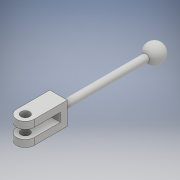
# Autodesk Inventor part: EndJoint
Saved by Autodesk Inventor 2018 (Build 220112000, 112)
## iProperties
Created: 2017-06-01
Part Number: EndJoint
Material: Generic
Document SubType Name: Modeling
Designer: Damian
Density: 1 g/cm^3
Appearance: Default
Author: Damian
Autodesk Inventor part; units mm, degrees
ref_plane "YZ Plane" through (0, 0, 0) normal (1, 0, 0) x (0, 1, 0)
ref_plane "XZ Plane" through (0, 0, 0) normal (0, 1, 0) x (-1, 0, 0)
ref_plane "XY Plane" through (0, 0, 0) normal (0, 0, 1) x (1, 0, 0)
sketch "Sketch1" plane through (0, 0, 0) normal (1, 0, 0) x (0, 1, 0)
  line L0 (0, 6.5) -> (24, 6.5)
  line L1 (24, 6.5) -> (24, -6.5)
  line L2 (24, -6.5) -> (0, -6.5)
  line L3 (0, -6.5) -> (0, -2.5)
  line L4 (0, -2.5) -> (20, -2.5)
  line L5 (20, -2.5) -> (20, 2.5)
  line L6 (20, 2.5) -> (0, 2.5)
  line L7 (0, 2.5) -> (0, 6.5)
  point P0 (0, 0)
  dimension "d0" = 4
  dimension "d1" = 20
  dimension "d2" = 4
  dimension "d3" = 5
  dimension "d11" = 2.5
  dimension "d12" = 0
  constraints: 16 end point, 7 perpendicular, 1 collinear, 1 horizontal, 1 point on line
  measures "d0" distance of L2.end L3.end
  measures "d1" distance of L3.end L4.end
  measures "d2" horizontal distance of L4.end L1.end
  measures "d3" distance of L4.end L5.end
  measures "d11" distance of L3.end point (0, 0)
  measures "d12" horizontal distance of point (0, 0) L3.end
extrude "Extrusion1" add sketch "Sketch1" along normal blind 10
sketch "Sketch2" plane through (0, 24, 6.5) normal (0, 1, 0) x (1, 0, 0)
  circle A0 centre (5, 6.5) radius 2
  line L0 (0, 0) -> (0, 13) projected
  line L1 (0, 13) -> (10, 13) projected
  point P0 (0, 6.5)
  dimension "d6" = 4
  dimension "d7" = 5
  dimension "d8" = 6.5
  constraints: 1 centre point
  measures "d6" diameter of A0
  measures "d7" distance from line of L0 A0.centre
  measures "d8" distance from line of L1 A0.centre
extrude "Extrusion2" add sketch "Sketch2" along normal blind 50
sketch "Sketch3" plane through (0, 0, 0) normal (0, 0, 1) x (1, 0, 0)
  line L0 (7, 74) -> (3, 74) projected
  line L1 (3, 74) -> (5, 74)
  line L2 (5, 74) -> (5, 84)
  arc A0 (5, 84) -> (3, 74) centre (5, 78.8) ccw
  point P0 (0, 0)
  dimension "d13" = 10
  constraints: 4 end point, 2 point on circle, 1 centre point, 1 midpoint, 1 perpendicular, 1 point on line
  measures "d13" distance of L1.end L2.end
revolve "Revolution1" add sketch "Sketch3" angle 360 about axis through (5, 74, 0) along (0, 1, 0)
fillet "Fillet1" radius 5 4 edges at (0, 0, -4.5) (10, 0, -4.5) (10, 0, 4.5) (0, 0, 4.5)
hole "Hole1" at (5, 5, -6.5) direction (0, 0, 1) diameter 5 end through all
body "Solid1"
